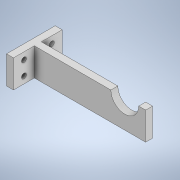
# Autodesk Inventor part: irrigationPipeSupport
Saved by Autodesk Inventor 2021.1 (Build 251245000, 245)
## iProperties
Created: 2020-09-15
Part Number: irrigationPipeSupport
Material: Generic
Document SubType Name: Modeling
Designer: robst
Density: 1 g/cm^3
Appearance: Default
Author: robst
Autodesk Inventor part; units mm, degrees
ref_plane "YZ Plane" through (0, 0, 0) normal (1, 0, 0) x (0, 1, 0)
ref_plane "XZ Plane" through (0, 0, 0) normal (0, 1, 0) x (-1, 0, 0)
ref_plane "XY Plane" through (0, 0, 0) normal (0, 0, 1) x (1, 0, 0)
sketch "Sketch2" plane through (0, 0, 0) normal (0, 0, 1) x (1, 0, 0)
  line L0 (0, 0) -> (107.95, 0)
  line L1 (107.95, 0) -> (107.95, 25.4)
  line L2 (0, 25.4) -> (0, 0)
  arc A0 (76.2, 25.4) -> (101.6, 25.4) centre (88.9, 25.4) ccw
  line L3 (107.95, 25.4) -> (101.6, 25.4)
  line L4 (76.2, 25.4) -> (0, 25.4)
  dimension "d0" = 107.95
  dimension "d1" = 25.4
  dimension "d2" = 25.4
  dimension "d3" = 88.9
  constraints: 10 end point, 3 parallel, 2 point on circle, 1 centre point, 1 horizontal, 1 perpendicular
  measures "d0" distance of L2.start L1.end
  measures "d1" distance of L1.end L0.end
  measures "d2" diameter of A0
  measures "d3" horizontal distance of A0.centre L0.start
extrude "Extrusion1" add sketch "Sketch2" along normal mid plane 6.35
sketch "Sketch3" plane through (0, 0, 0) normal (0, 0, 1) x (1, 0, 0)
  line L0 (0, 0) -> (0, 25.4) projected
  line L1 (0, 25.4) -> (76.2, 25.4) projected
  line L2 (107.95, 0) -> (0, 0) projected
  line L3 (0, 25.4) -> (6.35, 25.4)
  line L4 (6.35, 25.4) -> (6.35, 0)
  line L5 (6.35, 0) -> (0, 0)
  line L6 (0, 0) -> (0, 25.4)
  dimension "d17" = 6.35
  constraints: 8 end point, 2 parallel, 1 horizontal, 1 perpendicular, 1 point on line
  measures "d17" distance between parallel lines of L4 L0
extrude "Extrusion2" add sketch "Sketch3" along normal mid plane 44.45
sketch "Sketch4" plane through (6.35, 0, 3.175) normal (1, 0, 0) x (0, 0, -1)
  line L0 (-19.05, 0) -> (-19.05, 25.4) projected
  line L1 (-19.05, 25.4) -> (0, 25.4) projected
  line L2 (0, 0) -> (-19.05, 0) projected
  line L3 (0, 25.4) -> (0, 0) projected
  line L4 (-19.05, 25.4) -> (25.4, 25.4) construction
  line L5 (-9.525, 25.4) -> (-9.525, 0) construction
  point P0 (3.175, 0)
  point P1 (-9.525, 19.05)
  point P2 (-9.525, 6.35)
  dimension "d8" = 6.35
  dimension "d9" = 6.35
  constraints: 3 point on line, 2 end point, 1 midpoint
  measures "d8" distance from line of point (-9.525, 19.05) L1
  measures "d9" distance from line of point (-9.525, 6.35) L2
hole "Hole1" at (6.35, 19.05, 12.7) at (6.35, 6.35, 12.7) direction (-1, 0, 0) diameter 4.4958 end through all clearance for "Socket Head Cap Screw" size "#8" standard "Ansi Unified Screw Threads"
mirror "Mirror1" about plane through (0, 0, 0) normal (0, 0, 1) of "Hole1"
ref_plane "Work Plane1" through (0, 0, 0) normal (0, 0, 1) x (1, 0, 0)
equation "\"d0\" = supportLength"
equation "\"d1\" = supportHeight"
equation "\"d2\" = pipeDiameter"
equation "\"d3\" = distanceFromWallToPipeCenter"
equation "\"d4\" = supportWidth"
equation "\"d17\" = screwHoldDepth"
equation "\"d6\" = totalScrewHoldWidth"
equation "\"d8\" = screwPositionFromTop"
equation "\"d9\" = screwPositionFromTop"
equation "\"pipeDiameter\" = 25.4"
equation "\"distanceFromWallToPipeCenter\" = 88.9"
equation "\"supportLength\" = 107.95"
equation "\"supportHeight\" = 25.4"
equation "\"supportWidth\" = 6.35"
equation "\"screwHoldDepth\" = 6.35"
equation "\"screwHoldWidthExtension\" = 19.05"
equation "\"totalScrewHoldWidth\" = supportWidth + 2 * screwHoldWidthExtension"
equation "\"screwPositionFromTop\" = 6.35"
body "Solid1"
